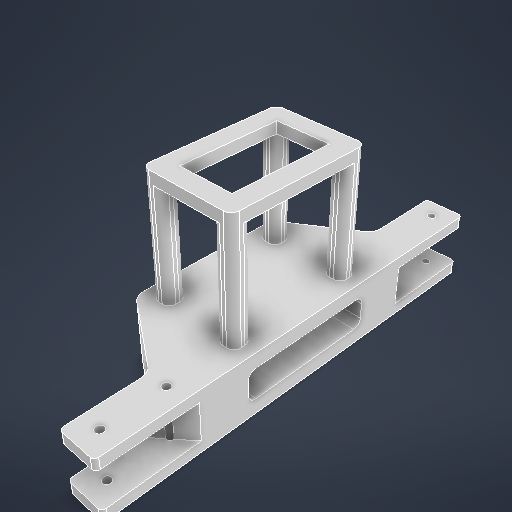
# Autodesk Inventor part: Front Bridge
Saved by Autodesk Inventor 2025 (Build 290162000, 162)
## iProperties
Created: 2024-05-23
Part Number: Front Bridge
Material: Generic
Document SubType Name: Modeling
Designer: DELL
Density: 1 g/cm^3
Appearance: Default
Author: DELL
Autodesk Inventor part; units mm, degrees
ref_plane "YZ Plane" through (0, 0, 0) normal (1, 0, 0) x (0, 1, 0)
ref_plane "XZ Plane" through (0, 0, 0) normal (0, 1, 0) x (-1, 0, 0)
ref_plane "XY Plane" through (0, 0, 0) normal (0, 0, 1) x (1, 0, 0)
sketch "Car Plan" plane through (0, 0, 0) normal (0, 1, 0) x (-1, 0, 0)
  line L0 (105, 0) -> (105, -20)
  line L1 (105, -20) -> (190, -20)
  line L2 (105, 0) -> (0, 0)
  line L3 (0, 0) -> (0, -96)
  line L4 (0, -96) -> (105, -96)
  line L5 (105, -96) -> (105, -76)
  line L6 (105, -76) -> (190, -76)
  line L7 (190, -76) -> (190, -20)
  line L8 (190, 32) -> (122, 32)
  line L9 (122, 32) -> (122, 5)
  line L10 (122, 5) -> (190, 5)
  line L11 (190, 5) -> (190, 32)
  line L12 (156, 5) -> (156, 0)
  line L13 (156, 0) -> (34, -48)
  point P0 (0, 32)
  point P1 (0, 32)
  point P2 (0, -48)
  dimension "d24" = 20
  dimension "d25" = 96
  dimension "d26" = 20
  dimension "d27" = 85
  dimension "d28" = 32
  dimension "d29" = 105
  dimension "d30" = 56
  dimension "d31" = 190
  dimension "d32" = 68
  dimension "d33" = 27
  dimension "d34" = 25
  dimension "d35" = 5
  dimension "d36" = 34
  dimension "d37" = 48
  constraints: 28 end point, 4 horizontal, 4 perpendicular, 3 vertical, 2 coincident, 2 collinear, 2 midpoint, 2 parallel, 1 point on line
  measures "d24" distance of L0.start L0.end
  measures "d25" distance of L2.end L3.end
  measures "d26" distance of L5.start L6.start
  measures "d27" distance between parallel lines of L0 L7
  measures "d28" distance from line of point (0, 32) L2
  measures "d29" distance between parallel lines of L3 L0
  measures "d30" distance from line of L6 L7.end
  measures "d31" distance between parallel lines of L3 L7
  measures "d32" distance of L10.end L9.end
  measures "d33" distance of L9.end L9.start
  measures "d34" distance between parallel lines of L1 L10
  measures "d35" distance of L12.start L12.end
  measures "d36" distance of point (0, -48) L13.end
  measures "d37" distance from line of L4 L13.end
sketch "Sketch5" plane through (0, 0, 0) normal (0, 1, 0) x (-1, 0, 0)
  line L0 (161, 5) -> (151, 5)
  line L1 (151, 5) -> (151, -101)
  line L2 (151, -101) -> (161, -101)
  line L3 (161, 5) -> (161, -15)
  line L4 (161, -101) -> (161, -81)
  line L5 (161, -15) -> (181, -28)
  line L6 (161, -15) -> (184.8537, -15) construction
  line L7 (161, -81) -> (181, -68)
  line L8 (161, -81) -> (184.8537, -81) construction
  line L9 (181, -68) -> (181, -28)
  point P0 (0, 0)
  point P1 (156, 0)
  point P2 (156, -96)
  dimension "d38" = 10
  dimension "d39" = 106
  dimension "d41" = 5
  dimension "d43" = 5
  dimension "d44" = 20
  dimension "d45" = 20
  dimension "d50" = 40
  dimension "d51" = 5
  dimension "d52" = 5
  dimension "d55" = 5
  dimension "d56" = 30
  constraints: 20 end point, 3 equal length, 3 horizontal, 2 perpendicular, 2 vertical, 1 parallel
  measures "d38" distance of L2.end L1.end
  measures "d39" distance of L1.end L0.end
  measures "d41" distance from line of L0 point (156, 0)
  measures "d43" distance from line of L2 point (156, -96)
  measures "d44" distance of L0.start L3.end
  measures "d45" distance of L2.end L4.end
  measures "d50" distance of L7.end L5.end
  measures "d51" distance from line of L3 point (156, 0)
  measures "d52" distance from line of L4 point (156, -96)
  measures "d55" distance from line of L1 point (156, 0)
  measures "d56" distance between parallel lines of L1 L9
extrude "Extrusion4" add sketch "Sketch5" along normal blind 16
sketch "Sketch6" plane through (-161, 0, 5) normal (0, 0, 1) x (1, 0, 0)
  line L0 (0, 0) -> (0, 16) projected
  line L1 (10, 0) -> (10, 16) projected
  line L2 (0, 13) -> (10, 13)
  line L3 (10, 13) -> (10, 3)
  line L4 (10, 3) -> (0, 3)
  line L5 (0, 3) -> (0, 13)
  line L6 (0, 16) -> (10, 16) projected
  line L7 (0, 0) -> (10, 0) projected
  point P0 (161, 0)
  point P1 (0, 3)
  point P2 (10, 13)
  dimension "d59" = 3
  dimension "d60" = 3
  constraints: 8 end point, 2 parallel, 2 point on line, 1 horizontal, 1 perpendicular
  measures "d59" distance between parallel lines of L6 L2
  measures "d60" distance between parallel lines of L7 L4
extrude "Extrusion5" cut sketch "Sketch6" against normal blind 15 contours L0 L2 L1 L4
sketch "Sketch7" plane through (0, 0, 0) normal (0, -1, 0) x (1, 0, 0)
  circle A0 centre (-156, -96) radius 1
  circle A1 centre (-156, 0) radius 1
  line L0 (-161, -15) -> (-161, 5) projected
  circle A2 centre (-156, -15) radius 1
  point P0 (0, 0)
  dimension "d63" = 2
  dimension "d64" = 2
  dimension "d126" = 15
  dimension "d127" = 5
  dimension "d128" = 2
  constraints: 3 centre point, 3 coincident
  measures "d63" diameter of A0
  measures "d64" diameter of A1
  measures "d126" distance of point (-156, -15) point (-156, 0)
  measures "d127" distance from line of L0 point (-156, -15)
  measures "d128" diameter of A2
extrude "Extrusion6" cut sketch "Sketch7" against normal through all
sketch "Sketch8" plane through (-151, 0, -101) normal (0, 0, -1) x (-1, 0, 0)
  line L0 (0, 13) -> (0, 3) projected
  line L1 (0, 3) -> (10, 3) projected
  line L2 (0, 13) -> (10, 13)
  line L3 (10, 13) -> (10, 3)
  line L4 (10, 3) -> (0, 3)
  line L5 (0, 3) -> (0, 13)
  point P0 (-151, 0)
  constraints: 8 end point, 2 parallel, 1 horizontal, 1 perpendicular
extrude "Extrusion7" cut sketch "Sketch8" against normal blind 15
sketch "Sketch9" plane through (-181, 0, -68) normal (-1, 0, 0) x (0, 0, 1)
  line L0 (3, 12) -> (37, 12)
  line L1 (37, 12) -> (37, 4)
  line L2 (37, 4) -> (3, 4)
  line L3 (3, 4) -> (3, 12)
  line L4 (0, 0) -> (0, 16) projected
  line L5 (40, 0) -> (40, 16) projected
  line L6 (0, 16) -> (40, 16) projected
  line L7 (0, 0) -> (40, 0) projected
  point P0 (68, 0)
  dimension "d72" = 3
  dimension "d73" = 3
  dimension "d76" = 4
  dimension "d77" = 4
  constraints: 8 end point, 2 parallel, 1 horizontal, 1 perpendicular
  measures "d72" distance between parallel lines of L3 L4
  measures "d73" distance between parallel lines of L5 L1
  measures "d76" distance between parallel lines of L6 L0
  measures "d77" distance between parallel lines of L7 L2
extrude "Extrusion8" cut sketch "Sketch9" against normal blind 30 contours L0 L1 L2 L3
fillet "Fillet1" radius 2 1 edges at (-166, 12, -65)
fillet "Fillet2" radius 2 1 edges at (-166, 12, -31)
fillet "Fillet7" radius 2 1 edges at (-166, 4, -65)
fillet "Fillet8" radius 2 1 edges at (-166, 4, -31)
sketch "Sketch11" plane through (0, 16, 0) normal (0, 1, 0) x (1, 0, 0)
  line L0 (-178, 30) -> (-173, 30)
  line L1 (-173, 30) -> (-173, 35)
  line L2 (-173, 35) -> (-178, 35)
  line L3 (-178, 35) -> (-178, 30)
  line L4 (-181, 68) -> (-181, 28) projected
  line L5 (-181, 28) -> (-161, 15) projected
  line L6 (-178, 61) -> (-173, 61)
  line L7 (-173, 61) -> (-173, 66)
  line L8 (-173, 66) -> (-178, 66)
  line L9 (-178, 66) -> (-178, 61)
  line L10 (-161, 81) -> (-181, 68) projected
  line L11 (-159, 30) -> (-154, 30)
  line L12 (-154, 30) -> (-154, 35)
  line L13 (-154, 35) -> (-159, 35)
  line L14 (-159, 35) -> (-159, 30)
  line L15 (-159, 61) -> (-154, 61)
  line L16 (-154, 66) -> (-159, 66)
  line L17 (-159, 66) -> (-159, 61)
  line L18 (-151, -5) -> (-151, 101) projected
  line L19 (-154, 61) -> (-154, 66)
  point P0 (0, 0)
  point P1 (-178, 32.5)
  point P2 (-175.5, 30)
  point P3 (-175.5, 66)
  dimension "d86" = 5
  dimension "d88" = 3
  dimension "d93" = 5
  dimension "d95" = 26
  dimension "d96" = 3
  dimension "d97" = 5
  dimension "d98" = 5
  dimension "d101" = 5
  dimension "d102" = 14
  dimension "d103" = 5
  dimension "d104" = 14
  dimension "d107" = 26
  dimension "d108" = 2
  dimension "d109" = 2
  dimension "d111" = 5
  constraints: 32 end point, 7 parallel, 4 horizontal, 4 perpendicular, 3 midpoint, 2 collinear
  measures "d86" distance of L2.end L1.end
  measures "d88" distance from line of L4 point (-178, 32.5)
  measures "d93" distance of L7.end L6.end
  measures "d95" distance between parallel lines of L2 L6
  measures "d96" distance between parallel lines of L4 L9
  measures "d97" distance of L6.start L6.end
  measures "d98" distance of L0.end L1.end
  measures "d101" distance of L13.end L12.end
  measures "d102" distance between parallel lines of L1 L14
  measures "d103" distance between parallel lines of L13 L11
  measures "d104" distance between parallel lines of L7 L17
  measures "d107" distance between parallel lines of L13 L15
  measures "d108" distance from line of L4.start L8
  measures "d109" distance from line of L4.end L0
  measures "d111" distance between parallel lines of L19 L17
extrude "Extrusion9" add sketch "Sketch11" along normal blind 28
sketch "Sketch12" plane through (0, 44, 0) normal (0, 1, 0) x (1, 0, 0)
  line L0 (-154, 30) -> (-159, 30) projected
  line L1 (-159, 61) -> (-159, 66) projected
  line L2 (-154, 30) -> (-159, 30)
  line L3 (-159, 30) -> (-159, 66)
  line L4 (-159, 66) -> (-154, 66)
  line L5 (-154, 66) -> (-154, 30)
  line L6 (-178, 30) -> (-178, 35) projected
  line L7 (-173, 61) -> (-173, 66) projected
  line L8 (-178, 30) -> (-173, 30)
  line L9 (-173, 30) -> (-173, 66)
  line L10 (-173, 66) -> (-178, 66)
  line L11 (-178, 66) -> (-178, 30)
  line L12 (-159, 35) -> (-154, 35) projected
  line L13 (-154, 35) -> (-178, 35)
  line L14 (-178, 35) -> (-178, 30)
  line L15 (-178, 30) -> (-154, 30)
  line L16 (-154, 30) -> (-154, 35)
  line L17 (-178, 61) -> (-173, 61) projected
  line L18 (-154, 66) -> (-178, 66)
  line L19 (-178, 66) -> (-178, 61)
  line L20 (-178, 61) -> (-154, 61)
  line L21 (-154, 61) -> (-154, 66)
  point P0 (0, 0)
  point P1 (-173, 35)
  constraints: 32 end point, 8 parallel, 4 horizontal, 4 perpendicular
extrude "Extrusion10" add sketch "Sketch12" along normal blind 3 contours L0 L3 L12 L5 | L15 L9 L13 L3 | L12 L3 L20 L5 | L8 L6 L13 L9 | L20 L1 L4 L5 | L20 L7 L18 L1 | L13 L11 L17 L9 | L17 L11 L10 L7
fillet "Fillet9" radius 2 1 edges at (-178, 31.5, -30)
fillet "Fillet10" radius 2 3 edges at (-178, 31.5, -66) (-154, 31.5, -30) (-154, 31.5, -66)
fillet "Fillet11" radius 2 11 edges at (-159, 30, -61) (-154, 30, -61) (-154, 30, -35) (-159, 30, -30) (-159, 30, -35) (-178, 30, -35) (-173, 30, -30) (-173, 30, -35) (-178, 30, -61) (-173, 30, -61) (-173, 30, -66)
fillet "Fillet12" radius 4 4 edges at (-181, 8, -68) (-181, 8, -28) (-161, 8, -15) (-161, 8, -81)
fillet "Fillet13" radius 1 8 edges at (-161, 14.5, 5) (-151, 14.5, 5) (-161, 1.5, 5) (-151, 1.5, 5) (-151, 14.5, -101) (-161, 14.5, -101) (-151, 1.5, -101) (-161, 1.5, -101)
sketch "Sketch14" plane through (-151, 0, -86) normal (0, 0, -1) x (-1, 0, 0)
  line L0 (10, 13) -> (10, 3) projected
  line L1 (0, 13) -> (10, 13) projected
  line L2 (10, 13) -> (-5, 13)
  line L3 (-5, 13) -> (-5, 3)
  line L4 (-5, 3) -> (10, 3)
  line L5 (10, 3) -> (10, 13)
  point P0 (-151, 0)
  dimension "d122" = 15
  constraints: 8 end point, 2 parallel, 1 horizontal, 1 perpendicular
  measures "d122" distance of L4.end L3.end
revolve "Revolution2" cut sketch "Sketch14" angle 40 about axis through (-161, 13, -86) along (0, -1, 0)
sketch "Sketch15" plane through (-161, 0, -10) normal (0, 0, 1) x (1, 0, 0)
  line L0 (0, 3) -> (0, 13) projected
  line L1 (0, 13) -> (15, 13)
  line L2 (15, 13) -> (15, 3)
  line L3 (15, 3) -> (0, 3)
  line L4 (0, 3) -> (0, 13)
  point P0 (161, 0)
  dimension "d124" = 15
  constraints: 8 end point, 2 parallel, 1 horizontal, 1 perpendicular
  measures "d124" distance of L2.end L3.end
revolve "Revolution3" cut sketch "Sketch15" angle 40 about axis through (-161, 3, -10) along (0, 1, 0)
body "Solid2"
